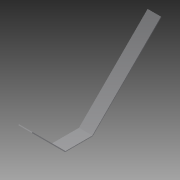
# Autodesk Inventor part: finger
Saved by Autodesk Inventor 2014 SP1 (Build 180222100, 222)
## iProperties
Created: 2013-11-11
Part Number: finger
Material: Polycarbonate, Clear
Document SubType Name: Modeling
Designer: RyanHughes
Density: 1.2 g/cm^3
Appearance: Polycarbonate - Clear
Author: RyanHughes
Autodesk Inventor part; units mm, degrees
note: some values were not read from the file. Chosen so that the rebuilt part matches the saved one: bend side of "Bend Part1"; bend side of "Bend Part2".
ref_plane "YZ Plane" through (0, 0, 0) normal (1, 0, 0) x (0, 1, 0)
ref_plane "XZ Plane" through (0, 0, 0) normal (0, 1, 0) x (-1, 0, 0)
ref_plane "XY Plane" through (0, 0, 0) normal (0, 0, 1) x (1, 0, 0)
sketch "Sketch1" plane through (0, 0, 0) normal (0, 1, 0) x (-1, 0, 0)
  line L0 (12.7, 161.925) -> (-12.7, 161.925)
  line L1 (-12.7, 161.925) -> (-12.7, -161.925)
  line L2 (-12.7, -161.925) -> (12.7, -161.925)
  line L3 (12.7, -161.925) -> (12.7, 161.925)
  line L4 (12.7, 161.925) -> (-12.7, -161.925) construction
  line L5 (-12.7, 161.925) -> (12.7, -161.925) construction
  point P0 (0, 0)
  dimension "d0" = 25.4
  dimension "d1" = 323.85
  constraints: 12 end point, 2 midpoint, 2 parallel, 1 horizontal, 1 perpendicular
  measures "d0" distance of L2.end L1.end
  measures "d1" distance of L1.end L0.end
extrude "Extrusion1" add sketch "Sketch1" along normal blind 1.5875
sketch "Sketch2" plane through (0, 1.5875, 0) normal (0, 1, 0) x (1, 0, 0)
  line L0 (-12.7, -161.925) -> (12.7, -161.925) projected
  line L1 (-43.2277, -22.225) -> (46.1542, -22.225)
  point P0 (0, 0)
  dimension "d4" = 139.7
  constraints: 2 end point
  measures "d4" distance between parallel lines of L0 L1
bend part "Bend Part1" radius 0.3234 angle 45 line through (-43.2277, 1.5875, 22.225) along (1, 0, 0) centre toward (0, 1, 0) moving side (0, 0, -1) both sides yes
sketch "Sketch4" plane through (-12.7, 1.6121, 22.3488) normal (0, 0.9238795, -0.3826834) x (1, 0, 0)
  line L0 (25.4, 0) -> (0, 0) projected
  line L1 (25.4, -139.573) -> (25.4, 0) projected
  line L2 (-18.5864, -50.8) -> (43.4016, -50.8)
  point P0 (12.7, 21.2645)
  dimension "d8" = 50.8
  constraints: 2 end point, 1 perpendicular
  measures "d8" distance between parallel lines of L0 L2
bend part "Bend Part2" radius 0.3234 angle 45 line through (-31.2864, 21.0524, 69.2818) along (1, 0, 0) centre toward (0, 0.9238795, -0.3826834) moving side (0, -0.3826834, -0.9238795) both sides yes
body "Solid1"
